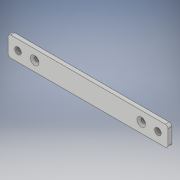
# Autodesk Inventor part: Power Supply Wall Mount v1
Saved by Autodesk Inventor 2019 (Build 230136000, 136)
## iProperties
Created: 2022-03-26
Part Number: Power Supply Wall Mount v1
Material: Generic
Document SubType Name: Modeling
Designer: Lix
Density: 1 g/cm^3
Appearance: Default
Author: Lix
Autodesk Inventor part; units mm, degrees
ref_plane "YZ Plane" through (0, 0, 0) normal (1, 0, 0) x (0, 1, 0)
ref_plane "XZ Plane" through (0, 0, 0) normal (0, 1, 0) x (-1, 0, 0)
ref_plane "XY Plane" through (0, 0, 0) normal (0, 0, 1) x (1, 0, 0)
sketch "Sketch1" plane through (0, 0, 0) normal (0, 0, 1) x (1, 0, 0)
  line L0 (-60, 7.5) -> (60, 7.5)
  line L1 (60, 7.5) -> (60, -7.5)
  line L2 (60, -7.5) -> (-60, -7.5)
  line L3 (-60, -7.5) -> (-60, 7.5)
  line L4 (-60, 7.5) -> (60, -7.5) construction
  line L5 (60, 7.5) -> (-60, -7.5) construction
  circle A0 centre (-52.5, 0) radius 2.5
  circle A1 centre (52.5, 0) radius 2.5
  point P0 (0, 0)
  point P1 (-60, 0)
  point P2 (60, 0)
  dimension "d0" = 120
  dimension "d1" = 15
  dimension "d2" = 5
  dimension "d3" = 7.5
  dimension "d4" = 7.5
  constraints: 12 end point, 4 midpoint, 2 centre point, 2 horizontal alignment, 2 parallel, 1 equal radius, 1 horizontal, 1 perpendicular
  measures "d0" distance of L1.end L2.end
  measures "d1" distance of L0.end L1.end
  measures "d2" diameter of A0
  measures "d3" distance from line of L3 A0.centre
  measures "d4" distance from line of L1 A1.centre
extrude "Extrusion1" add sketch "Sketch1" along normal blind 3
sketch "Sketch2" plane through (0, 0, 3) normal (0, 0, 1) x (1, 0, 0)
  line L0 (-40, 0) -> (40, 0) construction
  point P0 (0, 0)
  point P1 (0, 0)
  dimension "d7" = 80
  constraints: 2 end point, 2 horizontal alignment, 1 coincident, 1 horizontal, 1 midpoint
  measures "d7" distance of L0.start L0.end
hole "Hole1" at (-40, 0, 3) at (40, 0, 3) direction (0, 0, -1) diameter 3.3 depth 36.25 countersink diameter 6.5 countersink angle 90
fillet "Fillet1" radius 2 4 edges at (-60, 7.5, 1.5) (-60, -7.5, 1.5) (60, 7.5, 1.5) (60, -7.5, 1.5)
equation "\"d4\" = d3"
body "Solid1"
